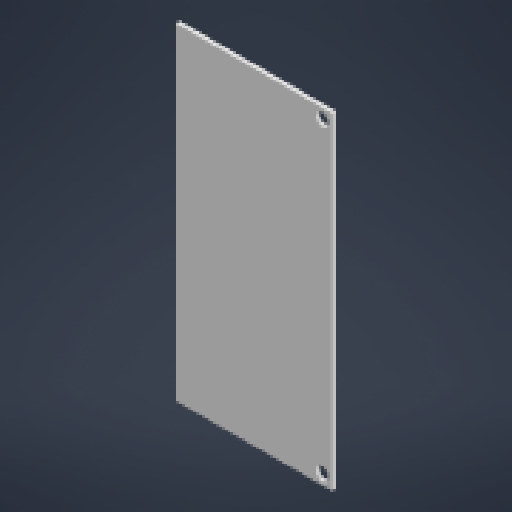
# Autodesk Inventor part: alert
Saved by Autodesk Inventor 2027.1 (Build 311270010, 270A)
## iProperties
Created: 2026-09-21
Part Number: alert
Material: Generic
Document SubType Name: Modeling
Designer: LENOVO
Density: 1 g/cm^3
Appearance: Default
Author: LENOVO
Autodesk Inventor part; units mm, degrees
ref_plane "YZ Plane" through (0, 0, 0) normal (1, 0, 0) x (0, 1, 0)
ref_plane "XZ Plane" through (0, 0, 0) normal (0, 1, 0) x (-1, 0, 0)
ref_plane "XY Plane" through (0, 0, 0) normal (0, 0, 1) x (1, 0, 0)
sketch "Sketch1" plane through (0, 0, 0) normal (0, 0, 1) x (1, 0, 0)
  line L0 (0, 0) -> (38.5, 0)
  line L1 (38.5, 0) -> (38.5, -80.7)
  line L2 (38.5, -80.7) -> (0, -80.7)
  line L3 (0, -80.7) -> (0, 0)
  circle A0 centre (36, -2.5) radius 1.6
  circle A1 centre (36, -78.2) radius 1.6
  dimension "d0" = 38.5
  dimension "d1" = 80.7
  dimension "d4" = 3.2
  dimension "d7" = 3.2
  constraints: 8 end point, 2 centre point, 2 parallel, 1 horizontal, 1 perpendicular
  measures "d0" distance of L1.end L2.end
  measures "d1" distance of L0.end L1.end
  measures "d4" diameter of A0
  measures "d7" diameter of A1
extrude "Extrusion1" add sketch "Sketch1" along normal blind 1
sketch "Sketch2" plane through (0, 0, 0) normal (0, 0, -1) x (-1, 0, 0)
  line L0 (0, -80.7) -> (-38.5, -80.7) projected
  line L1 (0, 0) -> (0, -80.7) projected
  line L2 (-38.5, 0) -> (0, 0) projected
  line L3 (-38.5, -80.7) -> (-38.5, 0) projected
  circle A0 centre (-36, -78.2) radius 1.6 projected
  circle A1 centre (-36, -2.5) radius 1.6 projected
  line L4 (-26.0363, 0) -> (-26.0363, -34.7)
  dimension "d10" = 34.7
  constraints: 2 end point, 1 point on line, 1 vertical
  measures "d10" distance of L4.start L4.end
body "Solid1"
